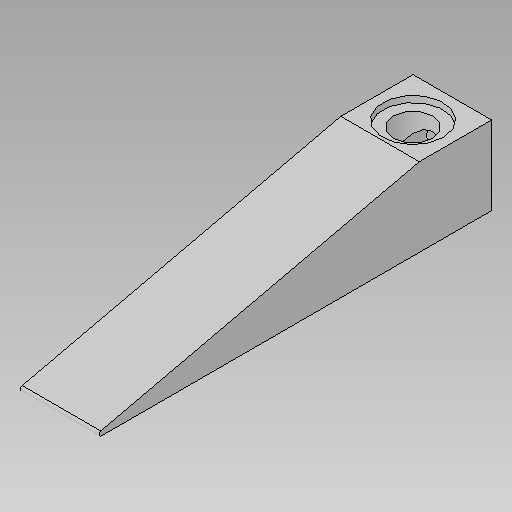
# Autodesk Inventor part: Wedge_base-single
Saved by Autodesk Inventor 2020 (Build 240168000, 168)
## iProperties
Created: 2019-02-07
Part Number: Wedge_base-single
Material: Generic
Document SubType Name: Modeling
Designer: Varga Daniel
Density: 1 g/cm^3
Appearance: Default
Author: Varga Daniel
Autodesk Inventor part; units mm, degrees
ref_plane "YZ Plane" through (0, 0, 0) normal (1, 0, 0) x (0, 1, 0)
ref_plane "XZ Plane" through (0, 0, 0) normal (0, 1, 0) x (-1, 0, 0)
ref_plane "XY Plane" through (0, 0, 0) normal (0, 0, 1) x (1, 0, 0)
derived "Connector_pin_base.ipt"
derived "Base_part.ipt"
sketch "Sketch2" plane through (0, 0, 0) normal (1, 0, 0) x (0, 1, 0)
  line L0 (0, 0) -> (10, 0)
  line L1 (10, 0) -> (10, 9.2)
  line L2 (10, 9.2) -> (0.5922, 49.7678)
  line L3 (0, 49.7) -> (0, 0)
  line L4 (0, 47.895) -> (8.9735, 9.2)
  line L5 (8.9735, 9.2) -> (0, 9.2)
  arc A0 (0.5922, 49.7678) -> (0, 49.7) centre (0.3, 49.7) ccw
  point P0 (0, 52.3216)
  dimension "d3" = 10
  dimension "d5" = 1
  dimension "d6" = 9.2
  dimension "d38" = 0.3
  dimension "d39" = 50
  constraints: 12 end point, 5 point on line, 2 parallel, 2 perpendicular, 2 point on circle, 2 tangent, 1 centre point, 1 horizontal
  measures "d3" distance between parallel lines of L1 L3
  measures "d5" distance between parallel lines of L2 L4
  measures "d6" distance between parallel lines of L5 L0
  measures "d38" radius of A0
extrude "Extrusion1" add sketch "Sketch2" against normal blind 10 contours L3 L5 L4 A0 L2 L1 L0
extrude "Left_wall" add sketch "Sketch2" against normal blind 1 contours L3 L4 L5
sketch "Sketch3" plane through (-10, 0, 0) normal (-1, 0, 0) x (0, 0, 1)
  line L0 (9.2, 8.9735) -> (9.2, 0) projected
  line L1 (47.895, 0) -> (9.2, 8.9735) projected
  line L2 (49.7, 0) -> (0, 0) projected
  point P0 (50, 0)
extrude "Right_wall" add sketch "Sketch3" against normal blind 1
sketch "Sketch4" plane through (-10, 0, 0) normal (0, -1, 0) x (1, 0, 0)
  line L0 (9, 47.895) -> (1, 47.895) construction
  line L1 (9, 9.2) -> (1, 9.2) construction
  line L2 (10, 0) -> (0, 0) construction
  circle A0 centre (5, 5) radius 3.85
  circle A1 centre (5, 5) radius 2.5
  line L3 (10, 49.7) -> (0, 49.7) projected
  line L4 (0, 0) -> (0, 49.7) projected
  line L5 (10, 49.7) -> (10, 0) projected
  line L6 (1, 47.895) -> (1, 9.2) projected
  line L7 (9, 9.2) -> (9, 47.895) projected
  dimension "d14" = 5
  dimension "d15" = 5
  dimension "d16" = 7.7
  dimension "d54" = 5
  constraints: 2 centre point, 1 coincident
  measures "d14" distance from line of A0.centre L2
  measures "d15" diameter of A1
  measures "d16" diameter of A0
  measures "d54" distance from line of A0.centre L4
extrude "Extrusion4" cut sketch "Sketch4" against normal through all contours A1
extrude "Extrusion6" cut sketch "Sketch4" against normal blind 0.8
sketch "Sketch6" plane through (0, 10, 9.2) normal (0, 1, 0) x (1, 0, 0)
  circle A0 centre (-5, 4.2) radius 3.85 projected
  circle A1 centre (-5, 4.2) radius 2.5 projected
  point P0 (0, 9.2)
extrude "Extrusion7" cut sketch "Sketch6" against normal blind 0.8
sketch "Sketch10" plane through (0, 0, 0) normal (0, 0, -1) x (-1, 0, 0)
  circle A0 centre (5, 5) radius 2.5
  circle A1 centre (5, 5) radius 3.85
  line L0 (0, 0) -> (0, 10) projected
  line L1 (0, 0) -> (10, 0) projected
  line L2 (10, 10) -> (10, 0) projected
  line L3 (0, 10) -> (10, 10) projected
  dimension "d43" = 5
  dimension "d44" = 7.7
  dimension "d55" = 5
  dimension "d56" = 5
  constraints: 2 centre point, 1 coincident
  measures "d43" diameter of A0
  measures "d44" diameter of A1
  measures "d55" distance from line of A0.centre L3
  measures "d56" distance from line of A0.centre L0
extrude "Extrusion11" cut sketch "Sketch10" against normal up to surface (9.2 mm away) contours A0
extrude "Extrusion12" cut sketch "Sketch10" against normal blind 0.8 contours A1
equation "\"d5\" = Wall_thickness"
equation "\"d6\" = 0.5 * Overall_height + 0.5 * Hole_height"
equation "\"d38\" = Wedge_end_fillet_radius"
equation "\"d39\" = Wedge_length"
equation "\"d9\" = Wall_thickness"
equation "\"d11\" = Wall_thickness"
equation "\"d15\" = Beam_hole_diameter"
equation "\"d16\" = Base_collar_diameter + Wedge_Pin_collar_diameter_tolerance"
equation "\"d24\" = -0.5 * Hole_height + 0.5 * Overall_height"
equation "\"d26\" = -0.5 * Hole_height + 0.5 * Overall_height"
equation "\"d43\" = Beam_hole_diameter"
equation "\"d44\" = Base_collar_diameter + Wedge_Pin_collar_diameter_tolerance"
equation "\"d50\" = -0.5 * Hole_height + 0.5 * Overall_height"
equation "\"Wedge_Pin_collar_diameter_tolerance\" = 0.2"
equation "\"Wedge_end_fillet_radius\" = 0.3"
equation "\"Wedge_wall_thickness\" = Wall_thickness"
equation "\"Wedge_fillet_radius\" = 0.3"
equation "\"Wall_thickness\" = 1"
equation "\"Overall_height\" = 10"
equation "\"Hole_height\" = 8.4"
equation "\"Wedge_length\" = 50"
equation "\"Beam_hole_diameter\" = 5"
equation "\"Base_collar_diameter\" = 7.5"
body "Solid1"
